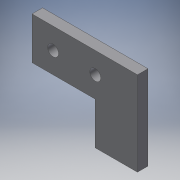
# Autodesk Inventor part: vrRig_v08_12inBreadboardStop
Saved by Autodesk Inventor 2016 (Build 200138000, 138)
## iProperties
Created: 2018-01-13
Part Number: vrRig_v08_12inBreadboardStop
Material: Generic
Document SubType Name: Modeling
Designer: harveylab
Density: 1 g/cm^3
Appearance: Default
Author: harveylab
Autodesk Inventor part; units mm, degrees
ref_plane "YZ Plane" through (0, 0, 0) normal (1, 0, 0) x (0, 1, 0)
ref_plane "XZ Plane" through (0, 0, 0) normal (0, 1, 0) x (-1, 0, 0)
ref_plane "XY Plane" through (0, 0, 0) normal (0, 0, 1) x (1, 0, 0)
sketch "Sketch1" plane through (0, 0, 0) normal (0, 0, 1) x (1, 0, 0)
  circle A0 centre (0, 0) radius 5.5 projected
  line L0 (12.6998, 0) -> (-114.3002, 0)
  line L1 (-114.3002, 0) -> (63.4998, 0)
  line L2 (63.4998, 0) -> (63.4998, -152.4)
  line L3 (63.4998, 0) -> (63.4998, 152.4)
  line L4 (63.4998, 152.4) -> (38.0998, 152.4)
  line L5 (63.4998, 152.4) -> (63.4998, 127)
  line L6 (63.4998, 127) -> (88.8998, 127)
  line L7 (88.8998, 127) -> (88.8998, 177.8)
  line L8 (88.8998, 177.8) -> (25.3998, 177.8)
  line L9 (25.3998, 177.8) -> (25.3998, 152.4)
  line L10 (25.3998, 152.4) -> (38.0998, 152.4)
  circle A1 centre (63.5, 165.1) radius 3.5 construction
  circle A2 centre (38.1, 165.1) radius 3.5 construction
  circle A3 centre (63.5, 165.1) radius 3.302
  circle A4 centre (38.1, 165.1) radius 3.302
  point P0 (0, 0)
  dimension "d0" = 127
  dimension "d1" = 177.8
  dimension "d2" = 152.4
  dimension "d3" = 152.4
  dimension "d4" = 25.4
  dimension "d5" = 25.4
  dimension "d6" = 25.4
  dimension "d7" = 50.8
  dimension "d8" = 63.5
  dimension "d11" = 6.604
  dimension "d12" = 6.604
  constraints: 22 end point, 7 perpendicular, 2 centre point, 2 coincident, 2 point on line, 1 horizontal, 1 vertical, 1 other
  measures "d0" distance of L0.start L0.end
  measures "d1" distance of L0.end L1.end
  measures "d2" distance of L1.end L2.end
  measures "d3" distance of L1.end L3.end
  measures "d4" distance of L3.end L4.end
  measures "d5" distance of L3.end L5.end
  measures "d6" distance of L5.end L6.end
  measures "d7" distance of L6.end L7.end
  measures "d8" distance of L7.end L8.end
  measures "d11" diameter of A3
  measures "d12" diameter of A4
extrude "Extrusion2" add sketch "Sketch1" along normal blind 6.35 contours L3 L4 L10 L9 L8 L7 L6
body "Solid2"
